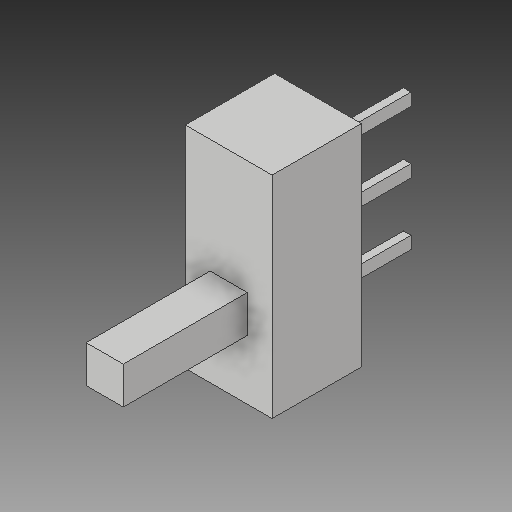
# Autodesk Inventor part: Circuit_SlideSwitch_SS-12D00-G5
Saved by Autodesk Inventor 2018.2 (Build 222227000, 227)
## iProperties
Created: 2017-09-29
Part Number: Circuit_SlideSwitch_SS-12D00-G5
Material: 一般
Document SubType Name: Modeling
Designer: sktom
Density: 1 g/cm^3
Appearance: 既定
Author: sktom
Title: Circuit_SlideSwitch_SS-12D00-G5
Autodesk Inventor part; units mm, degrees
ref_plane "YZ Plane" through (0, 0, 0) normal (1, 0, 0) x (0, 1, 0)
ref_plane "XZ Plane" through (0, 0, 0) normal (0, 1, 0) x (-1, 0, 0)
ref_plane "XY Plane" through (0, 0, 0) normal (0, 0, 1) x (1, 0, 0)
sketch "スケッチ1" plane through (0, 0, 0) normal (0, 0, 1) x (1, 0, 0)
  line L0 (-1.75, -4.25) -> (1.75, -4.25)
  line L1 (1.75, -4.25) -> (1.75, 4.25)
  line L2 (1.75, 4.25) -> (-1.75, 4.25)
  line L3 (-1.75, 4.25) -> (-1.75, -4.25)
  line L4 (-1.75, -4.25) -> (1.75, 4.25) construction
  line L5 (1.75, -4.25) -> (-1.75, 4.25) construction
  point P0 (0, 0)
  dimension "d0" = 8.5
  dimension "d1" = 3.5
  constraints: 12 end point, 2 midpoint, 2 parallel, 1 horizontal, 1 perpendicular
  measures "d0" distance of L0.end L1.end
  measures "d1" distance of L1.end L2.end
extrude "押し出し1" add sketch "スケッチ1" along normal blind 3.6
sketch "スケッチ2" plane through (0, 0, 3.6) normal (0, 0, 1) x (1, 0, 0)
  line L0 (-0.75, 1.85) -> (0.75, 1.85) construction
  line L1 (0.75, 1.85) -> (0.75, -1.85) construction
  line L2 (0.75, -1.85) -> (-0.75, -1.85) construction
  line L3 (-0.75, -1.85) -> (-0.75, 1.85) construction
  line L4 (-0.75, 1.85) -> (0.75, -1.85) construction
  line L5 (0.75, 1.85) -> (-0.75, -1.85) construction
  line L6 (-0.75, -1.85) -> (0.75, -1.85)
  line L7 (0.75, -1.85) -> (0.75, -0.35)
  line L8 (0.75, -0.35) -> (-0.75, -0.35)
  line L9 (-0.75, -0.35) -> (-0.75, -1.85)
  point P0 (0, 0)
  dimension "d4" = 3.7
  dimension "d5" = 1.5
  dimension "d6" = 1.5
  constraints: 20 end point, 4 parallel, 2 horizontal, 2 midpoint, 2 perpendicular, 1 point on line
  measures "d4" distance of L0.end L1.end
  measures "d5" distance of L0.start L0.end
  measures "d6" distance between parallel lines of L2 L8
extrude "押し出し2" add sketch "スケッチ2" along normal blind 5
sketch "スケッチ3" plane through (0, 0, 0) normal (0, 0, -1) x (-1, 0, 0)
  line L0 (-0.15, -2.75) -> (0.15, -2.75) construction
  line L1 (0.15, -2.75) -> (0.15, 2.75) construction
  line L2 (0.15, 2.75) -> (-0.15, 2.75) construction
  line L3 (-0.15, 2.75) -> (-0.15, -2.75) construction
  line L4 (-0.15, -2.75) -> (0.15, 2.75) construction
  line L5 (0.15, -2.75) -> (-0.15, 2.75) construction
  line L6 (-0.15, 2.75) -> (0.15, 2.75)
  line L7 (0.15, 2.75) -> (0.15, 2.25)
  line L8 (0.15, 2.25) -> (-0.15, 2.25)
  line L9 (-0.15, 2.25) -> (-0.15, 2.75)
  line L10 (-0.15, -0.25) -> (0.15, -0.25)
  line L11 (0.15, -0.25) -> (0.15, 0.25)
  line L12 (0.15, 0.25) -> (-0.15, 0.25)
  line L13 (-0.15, 0.25) -> (-0.15, -0.25)
  line L14 (-0.15, -0.25) -> (0.15, 0.25) construction
  line L15 (0.15, -0.25) -> (-0.15, 0.25) construction
  line L16 (-0.15, -2.75) -> (0.15, -2.75)
  line L17 (0.15, -2.75) -> (0.15, -2.25)
  line L18 (0.15, -2.25) -> (-0.15, -2.25)
  line L19 (-0.15, -2.25) -> (-0.15, -2.75)
  point P0 (0, 0)
  dimension "d9" = 0.3
  dimension "d10" = 5.5
  dimension "d11" = 0.5
  dimension "d12" = 0.5
  dimension "d13" = 0.5
  constraints: 40 end point, 8 parallel, 4 horizontal, 4 midpoint, 4 perpendicular, 3 point on line
  measures "d9" distance of L1.end L2.end
  measures "d10" distance of L0.end L1.end
  measures "d11" distance of L6.end L7.end
  measures "d12" distance between parallel lines of L10 L12
  measures "d13" distance between parallel lines of L0 L18
extrude "押し出し3" add sketch "スケッチ3" along normal blind 3.6
